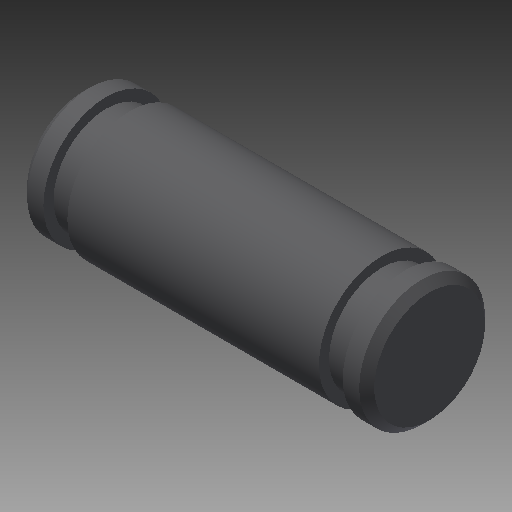
# Autodesk Inventor part: D-8381
Saved by Autodesk Inventor 2017 (Build 210142000, 142)
## iProperties
Category: PARTsolutions
Company: BIMBA
Created: 2016-11-12
Part Number: D-8381
Catalog Web Link: www.cadenas.de
Description: Piston Rod Clevis for Original Line Cylinders - Pin-
Vendor: BIMBA
Document SubType Name: Modeling
Designer: psAdmin
Manufacturer: BIMBA
Mass: 0.529757 g
Surface Area: 4.33276 cm^2
Volume: 0.529757 cm^3
Density: 1 g/cm^3
Material: Generic
Appearance: PSOLRGB-191-191-191
PSOL_IDENT_0: {$CADENAS_DATA\23d-libs\bimba\bimba\bimba_imperial\bimba_full_line\original_line_cylinders\accessori
PSOL_IDENT_1: es\piston_rod_clevis_pin.prj},199 {VTYP=3D},{NB=D-8381},{LINA=D-8381},{NN=Piston Rod Clevis for Orig
PSOL_IDENT_2: inal Line Cylinders - Pin},{DATE=09.11.2016 07:55:10},{GEOMDATE=03.04.2013 12:23:00},{VERSION=},{LIN
PSOL_IDENT_3: EID=30},{LINESUBID=-1},{WBVAR=}  {NB=D-8381},{LINA=D-8381},{KT=DUMMY},{PN=D-8381},{L=0.69000000},{L1=
PSOL_IDENT_4: 0.50000000},{L2=0.04750000},{L4=0.04750000},{D=0.25000000},{D1=0.21000000},{CH=0.01500000},{R=0.0025
PSOL_IDENT_5: 0000},{COLOR=0.75,0.75,0.75,0.00}
NN: Piston Rod Clevis for Original Line Cylinders - Pin
NB: D-8381
NBSYN: $PN.
LINA: D-8381
PN: D-8381
L: 0.69000000
L1: 0.50000000
L2: 0.04750000
L4: 0.04750000
D: 0.25000000
D1: 0.21000000
CH: 0.01500000
R: 0.00250000
SUPPLIER: BIMBA
ARTICLENO: D-8381
BOMINFO: D-8381
CREATOR: CADENAS GmbH
Title: D-8381
Author: Cadenas PARTsolutions
Autodesk Inventor part; units mm, degrees
sketch "Sketch_1" plane through (0, 0, 0) normal (0, 0, 1) x (1, 0, 0)
  line L0 (8.763, 0) -> (-8.763, 0)
  line L1 (-8.763, 0) -> (-8.763, 2.794)
  line L2 (-8.763, 2.794) -> (-8.382, 3.175)
  line L3 (-8.382, 3.175) -> (-7.5565, 3.175)
  line L4 (-7.5565, 3.175) -> (-7.5565, 2.667)
  line L5 (-7.5565, 2.667) -> (-6.35, 2.667)
  line L6 (-6.35, 2.667) -> (-6.35, 3.175)
  line L7 (-6.35, 3.175) -> (6.35, 3.175)
  line L8 (6.35, 3.175) -> (6.35, 2.667)
  line L9 (6.35, 2.667) -> (7.5565, 2.667)
  line L10 (7.5565, 2.667) -> (7.5565, 3.175)
  line L11 (7.5565, 3.175) -> (8.382, 3.175)
  line L12 (8.382, 3.175) -> (8.763, 2.794)
  line L13 (8.763, 2.794) -> (8.763, 0)
  line L14 (8.763, 0) -> (-8.763, 0)
  constraints: 30 end point
revolve "Revolution1" add sketch "Sketch_1" angle 360 about axis through (8.763, 0, 0) along (1, 0, 0)
ref_plane "p1_XY" through (0, 0, 3.175) normal (1, 0, 0) x (0, 0, -1)
ref_plane "p1_YZ" through (0, 0, 3.175) normal (0, 0, -1) x (0, 1, 0)
ref_plane "p1_ZX" through (0, 0, 3.175) normal (0, 1, 0) x (1, 0, 0)
ref_plane "p2_XY" through (0, 0, -3.175) normal (1, 0, 0) x (0, 0, -1)
ref_plane "p2_YZ" through (0, 0, -3.175) normal (0, 0, -1) x (0, 1, 0)
ref_plane "p2_ZX" through (0, 0, -3.175) normal (0, 1, 0) x (1, 0, 0)
ref_plane "pin_XY" through (0, 0, 0) normal (1, 0, 0) x (0, 0, -1)
ref_plane "pin_YZ" through (0, 0, 0) normal (0, 0, -1) x (0, 1, 0)
ref_plane "pin_ZX" through (0, 0, 0) normal (0, 1, 0) x (1, 0, 0)
ref_plane "rr1_XY" through (6.9532, 0, 0) normal (1, 0, 0) x (0, 0, -1)
ref_plane "rr1_YZ" through (6.9532, 0, 0) normal (0, 0, -1) x (0, 1, 0)
ref_plane "rr1_ZX" through (6.9532, 0, 0) normal (0, 1, 0) x (1, 0, 0)
ref_plane "rr2_XY" through (-6.9532, 0, 0) normal (1, 0, 0) x (0, 0, -1)
ref_plane "rr2_YZ" through (-6.9532, 0, 0) normal (0, 0, -1) x (0, 1, 0)
ref_plane "rr2_ZX" through (-6.9532, 0, 0) normal (0, 1, 0) x (1, 0, 0)
ref_plane "w21_XY" through (8.763, 0, 0) normal (0, 1, 0) x (1, 0, 0)
ref_plane "w21_YZ" through (8.763, 0, 0) normal (1, 0, 0) x (0, 0, -1)
ref_plane "w21_ZX" through (8.763, 0, 0) normal (0, 0, -1) x (0, 1, 0)
ref_plane "w22_XY" through (-8.763, 0, 0) normal (0, 1, 0) x (1, 0, 0)
ref_plane "w22_YZ" through (-8.763, 0, 0) normal (1, 0, 0) x (0, 0, -1)
ref_plane "w22_ZX" through (-8.763, 0, 0) normal (0, 0, -1) x (0, 1, 0)
body "Solid1"
